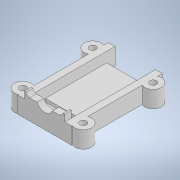
# Autodesk Inventor part: motor_top
Saved by Autodesk Inventor 2020.4 (Build 244396000, 396)
## iProperties
Created: 2020-08-20
Part Number: motor_top
Material: Generic
Document SubType Name: Modeling
Designer: Tarsoly
Density: 1 g/cm^3
Appearance: Default
Author: Tarsoly
Autodesk Inventor part; units mm, degrees
ref_plane "YZ Plane" through (0, 0, 0) normal (1, 0, 0) x (0, 1, 0)
ref_plane "XZ Plane" through (0, 0, 0) normal (0, 1, 0) x (-1, 0, 0)
ref_plane "XY Plane" through (0, 0, 0) normal (0, 0, 1) x (1, 0, 0)
sketch "Sketch1" plane through (0, 0, 0) normal (0, 1, 0) x (-1, 0, 0)
  line L0 (8, 13.5) -> (-8, 13.5)
  line L1 (-8, 13.5) -> (-8, -13.5)
  line L2 (-8, -13.5) -> (8, -13.5)
  line L3 (8, -13.5) -> (8, 13.5)
  line L4 (8, 13.5) -> (-8, -13.5) construction
  line L5 (-8, 13.5) -> (8, -13.5) construction
  point P0 (0, 0)
  dimension "d0" = 16
  dimension "d1" = 27
  constraints: 12 end point, 2 midpoint, 2 parallel, 1 horizontal, 1 perpendicular
  measures "d0" distance of L0.start L0.end
  measures "d1" distance of L2.end L0.start
extrude "Extrusion1" add sketch "Sketch1" along normal blind 2
sketch "Sketch2" plane through (0, 2, 0) normal (0, 1, 0) x (1, 0, 0)
  line L0 (8, 13.5) -> (-8, 13.5) projected
  line L1 (-6, 13.5) -> (6, 13.5)
  line L2 (6, 13.5) -> (6, -11.5)
  line L3 (6, -11.5) -> (-6, -11.5)
  line L4 (-6, -11.5) -> (-6, 13.5)
  line L5 (8, -13.5) -> (8, 13.5) projected
  line L6 (-8, 13.5) -> (-8, -13.5) projected
  line L7 (-8, -13.5) -> (8, -13.5) projected
  point P0 (0, 0)
  dimension "d4" = 2
  dimension "d5" = 2
  dimension "d6" = 2
  constraints: 8 end point, 2 parallel, 1 horizontal, 1 perpendicular, 1 point on line
  measures "d4" distance between parallel lines of L5 L2
  measures "d5" distance between parallel lines of L6 L4
  measures "d6" distance between parallel lines of L7 L3
extrude "Extrusion2" add sketch "Sketch2" along normal blind 3 contours L5 L7 L6 L0 L4 L3 L2
sketch "Sketch4" plane through (0, 5, 0) normal (0, 1, 0) x (1, 0, 0)
  line L0 (6, -11.5) -> (-6, -11.5) projected
  line L1 (-8, -13.5) -> (8, -13.5) projected
  line L2 (-6, -11.5) -> (6, -11.5)
  line L3 (6, -11.5) -> (6, -13.5)
  line L4 (6, -13.5) -> (-6, -13.5)
  line L5 (-6, -13.5) -> (-6, -11.5)
  line L6 (6, 13.5) -> (6, -11.5) projected
  point P0 (0, 0)
  constraints: 8 end point, 2 parallel, 1 collinear, 1 horizontal, 1 perpendicular, 1 point on line
extrude "Extrusion3" add sketch "Sketch4" along normal blind 2
sketch "Sketch3" plane through (-8, 0, 13.5) normal (0, 0, 1) x (1, 0, 0)
  line L0 (14, 2) -> (2, 2) construction
  line L1 (2, 2) -> (14, 2) construction
  circle A0 centre (8, 7) radius 2.5
  line L2 (8, 11.4) -> (8, -1.9) construction
  line L3 (3.5, 7) -> (12.5, 7) construction
  circle A1 centre (3.5, 7) radius 1
  circle A2 centre (12.5, 7) radius 1
  line L4 (3.5, 8) -> (5.7087, 8)
  line L5 (12.5, 8) -> (10.2913, 8)
  line L6 (12.5, 6) -> (10.2913, 6)
  line L7 (5.7087, 6) -> (3.5, 6)
  point P0 (8, 0)
  dimension "d9" = 5
  dimension "d10" = 5
  dimension "d11" = 9
  dimension "d12" = 2
  dimension "d13" = 2
  constraints: 10 end point, 8 point on circle, 4 point on line, 3 centre point, 3 horizontal, 3 tangent, 2 coincident, 2 midpoint, 1 parallel
  measures "d9" distance from line of L0 A0.centre
  measures "d10" diameter of A0
  measures "d11" distance of L3.start L3.end
  measures "d12" diameter of A2
  measures "d13" diameter of A1
extrude "Extrusion4" cut sketch "Sketch3" against normal up to next
sketch "Sketch8" plane through (0, 2, 0) normal (0, 1, 0) x (1, 0, 0)
  line L0 (-6, 13.5) -> (-6, -11.5) projected
  line L1 (6, -11.5) -> (6, 13.5) projected
  line L2 (-6, 13.5) -> (6, 13.5)
  line L3 (6, 13.5) -> (6, 11)
  line L4 (6, 11) -> (-6, 11)
  line L5 (-6, 11) -> (-6, 13.5)
  line L6 (-2.2913, -11.5) -> (2.2913, -11.5) projected
  point P0 (0, 0)
  point P1 (6, 13.5)
  point P2 (-6, 11)
  dimension "d28" = 22.5
  constraints: 8 end point, 2 parallel, 1 horizontal, 1 perpendicular, 1 point on line
  measures "d28" distance between parallel lines of L6 L4
extrude "Extrusion7" cut sketch "Sketch8" against normal up to next
sketch "Sketch9" plane through (0, 2, 0) normal (0, 1, 0) x (1, 0, 0)
  line L0 (-6, 11) -> (-6, -11.5) projected
  line L1 (6, -11.5) -> (6, 11) projected
  line L2 (-6, -10.5) -> (6, -10.5)
  line L3 (6, -10.5) -> (6, -7.3)
  line L4 (6, -7.3) -> (-6, -7.3)
  line L5 (-6, -7.3) -> (-6, -10.5)
  line L6 (-2.2913, -11.5) -> (2.2913, -11.5) projected
  point P0 (0, 0)
  point P1 (6, -10.5)
  dimension "d31" = 1
  dimension "d32" = 3.2
  constraints: 8 end point, 2 parallel, 2 point on line, 1 horizontal, 1 perpendicular
  measures "d31" distance between parallel lines of L6 L2
  measures "d32" distance between parallel lines of L2 L4
extrude "Extrusion8" cut sketch "Sketch9" against normal blind 1
sketch "Sketch10" plane through (0, 0, 0) normal (0, -1, 0) x (1, 0, 0)
  circle A0 centre (-9, 11) radius 1
  circle A1 centre (-9, 11) radius 2.5
  line L0 (-8, -13.5) -> (-8, 13.5) projected
  line L1 (-8, 13.5) -> (8, 13.5) projected
  line L2 (8, 13.5) -> (8, -13.5) projected
  line L3 (-8, 13.5) -> (-6, 13.5) projected
  circle A2 centre (-9, -9.8) radius 1
  circle A3 centre (-9, -9.8) radius 2.5
  circle A4 centre (9, 11) radius 1
  circle A5 centre (9, 11) radius 2.5
  circle A6 centre (9, -9.8) radius 1
  circle A7 centre (9, -9.8) radius 2.5
  point P0 (0, 0)
  point P1 (-8, -7.3)
  point P2 (10, 13.5)
  point P3 (10, -7.3)
  point P4 (-8, 11)
  point P5 (-8, 13.2913)
  point P6 (-8, 8.7087)
  point P7 (-8, -7.5087)
  point P8 (-8, -12.0913)
  point P9 (-8, -9.8)
  point P10 (8, 13.2913)
  point P11 (8, 11)
  point P12 (8, 8.7087)
  dimension "d35" = 2
  dimension "d36" = 1.5
  dimension "d37" = 27
  dimension "d38" = 16
  dimension "d41" = 20.8
  dimension "d44" = 18
  constraints: 8 centre point, 2 tangent, 1 horizontal, 1 vertical, 12 other
  measures "d35" diameter of A0
  measures "d36" radial gap between concentric circles of A0 A1
  measures "d37" distance of L0.start L0.end
  measures "d38" distance of L0.end L1.end
  measures "d41" distance of A0.centre A2.centre
  measures "d44" distance of A0.centre A4.centre
extrude "Extrusion9" add sketch "Sketch10" against normal up to surface (5 mm away) contours L0 A1 | A3 L0 | A5 L2 | A7 L2 | L2 A7 picked at (-10.9649, 10.7158) picked at (-10.9649, -10.0842) picked at (10.9649, 10.7158)
equation "\"d5\" = d4"
equation "\"d6\" = d4"
body "Solid1"
